Shaft_v4 (Autodesk Fusion 360 design; units mm, degrees)
Autodesk Fusion 360 part; units mm, degrees
sketch "Esquisse1" plane through (0, 0, 0) normal (0, 0, 1) x (1, 0, 0) in component "threaded shaft"
  circle A0 centre (0, 0) radius 2.5
  dimension "d1" = 5
  constraint coincident A0.centre origin
  measures "d1" diameter of A0
extrude "Extrusion1" add sketch "Esquisse1" along normal blind 337 makes body 1 in component "threaded shaft"
thread "Filetage1" "ISO Metric profile 5.0 M5x0.8 6g" major diameter 4.901 minor diameter 3.9895 pitch 0.8 angle 60 resizes the face on face at (2.4905, -0.2179, 224.6667) on bodies 1 in component "threaded shaft"
sketch "Esquisse2" plane through (0, 0, 0) normal (0, 0, 1) x (1, 0, 0) in component "Bolt"
  circle A0 centre (0, 0) radius 2.5
  circle A1 centre (0, 0) radius 4 construction
  line L0 (4, 2.3094) -> (0, 4.6188)
  line L1 (0, 4.6188) -> (-4, 2.3094)
  line L2 (-4, 2.3094) -> (-4, -2.3094)
  line L3 (-4, -2.3094) -> (0, -4.6188)
  line L4 (0, -4.6188) -> (4, -2.3094)
  line L5 (4, -2.3094) -> (4, 2.3094)
  dimension "d4" = 5
  dimension "d5" = 8
  dimension "d6" = 8
  constraint coincident A0.centre A1.centre
  constraint concentric A0 A1
  constraint vertical L2
  measures "d4" diameter of A0
  measures "d5" diameter of A1
  measures "d6" distance of L1 L4
extrude "Extrusion2" add sketch "Esquisse2" along normal blind 4 separate body makes body 2 in component "Bolt"
copy_body "CutPasteBodies1" bodies 2 removing the originals makes body 3 in component "Bolt"
thread "Filetage1'" "ISO Metric profile 5.0 M5x0.8 6H" major diameter 5.12 minor diameter 4.234 pitch 0.8 angle 60 resizes the face on face at (2.4969, -0.1246, 2.6667) on bodies 3 in component "Bolt"
component "threaded shaft" placed x (1, 0, 0) y (0, 1, 0) z (0, 0, 1) at (0, 0, 0)
component "Bolt" placed x (1, 0, 0) y (0, 1, 0) z (0, 0, 1) at (0, 0, 0)
component "Bolt" placed x (1, 0, 0) y (0, 1, 0) z (0, 0, 1) at (0, 0, 333)
equation "d6 = d5"
